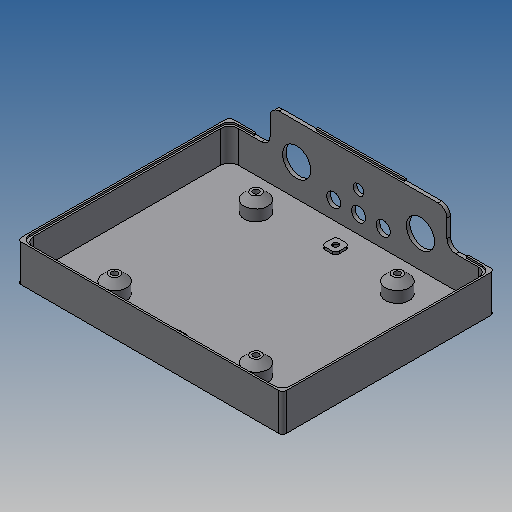
# Autodesk Inventor part: Base_Meca_IIm_Ligne
Saved by Autodesk Inventor 2025.3 (Build 293356000, 356)
## iProperties
Created: 2026-08-21
Part Number: Base_Meca_IIm_Ligne
Project: Nom Projet
Material: .
Description: Nom pièce
Document SubType Name: Modeling
Designer: jules
Authority: brut Ø
Density: 0.001 g/cm^3
Appearance: Par défaut
Mass: 0.0628592 g
Surface Area: 622.043 cm^2
Volume: 62.8592 cm^3
Material number: ---
Author: jules
Autodesk Inventor part; units mm, degrees
ref_plane "Plan YZ" through (0, 0, 0) normal (1, 0, 0) x (0, 1, 0)
ref_plane "Plan XZ" through (0, 0, 0) normal (0, 1, 0) x (-1, 0, 0)
ref_plane "Plan XY" through (0, 0, 0) normal (0, 0, 1) x (1, 0, 0)
sketch "Esquisse1" plane through (0, 0, 0) normal (0, 0, 1) x (1, 0, 0)
  line L0 (40, -40) -> (-40, -40) construction
  line L1 (-40, -40) -> (-40, 40) construction
  line L2 (-40, 40) -> (40, 40) construction
  line L3 (40, 40) -> (40, -40) construction
  line L4 (40, -40) -> (-40, 40) construction
  line L5 (-40, -40) -> (40, 40) construction
  line L6 (75, -60) -> (-75, -60)
  line L7 (-75, -60) -> (-75, 60)
  line L8 (-75, 60) -> (75, 60)
  line L9 (75, 60) -> (75, -60)
  line L10 (75, -60) -> (-75, 60) construction
  line L11 (-75, -60) -> (75, 60) construction
  line L12 (-36.8246, 40) -> (-38.4123, 37.25)
  line L13 (-38.4123, 37.25) -> (-41.5877, 37.25)
  line L14 (-41.5877, 37.25) -> (-43.1754, 40)
  line L15 (-43.1754, 40) -> (-41.5877, 42.75)
  line L16 (-41.5877, 42.75) -> (-38.4123, 42.75)
  line L17 (-38.4123, 42.75) -> (-36.8246, 40)
  line L18 (0, -84) -> (0, 84) construction
  line L19 (-105, 0) -> (105, 0) construction
  circle A0 centre (-40, 40) radius 1.75 construction
  circle A1 centre (-40, 40) radius 6.75
  line L20 (43.1754, 40) -> (41.5877, 37.25)
  line L21 (41.5877, 42.75) -> (43.1754, 40)
  line L22 (38.4123, 42.75) -> (41.5877, 42.75)
  line L23 (36.8246, 40) -> (38.4123, 42.75)
  line L24 (38.4123, 37.25) -> (36.8246, 40)
  line L25 (41.5877, 37.25) -> (38.4123, 37.25)
  circle A2 centre (40, 40) radius 6.75
  line L26 (-36.8246, -40) -> (-38.4123, -42.75)
  line L27 (-38.4123, -37.25) -> (-36.8246, -40)
  line L28 (-41.5877, -37.25) -> (-38.4123, -37.25)
  line L29 (-43.1754, -40) -> (-41.5877, -37.25)
  line L30 (-41.5877, -42.75) -> (-43.1754, -40)
  line L31 (-38.4123, -42.75) -> (-41.5877, -42.75)
  circle A3 centre (-40, -40) radius 6.75
  line L32 (43.1754, -40) -> (41.5877, -42.75)
  line L33 (41.5877, -37.25) -> (43.1754, -40)
  line L34 (38.4123, -37.25) -> (41.5877, -37.25)
  line L35 (36.8246, -40) -> (38.4123, -37.25)
  line L36 (38.4123, -42.75) -> (36.8246, -40)
  line L37 (41.5877, -42.75) -> (38.4123, -42.75)
  circle A4 centre (40, -40) radius 6.75
  circle A5 centre (0, 45.025) radius 1.6 construction
  circle A6 centre (0, -45.025) radius 1.6 construction
  line L38 (-2.75, 46.6127) -> (0, 48.2004)
  line L39 (0, 48.2004) -> (2.75, 46.6127)
  line L40 (2.75, 46.6127) -> (2.75, 43.4373)
  line L41 (2.75, 43.4373) -> (0, 41.8496)
  line L42 (0, 41.8496) -> (-2.75, 43.4373)
  line L43 (-2.75, 43.4373) -> (-2.75, 46.6127)
  line L44 (-2.75, -46.6127) -> (0, -48.2004)
  line L45 (0, -48.2004) -> (2.75, -46.6127)
  line L46 (2.75, -46.6127) -> (2.75, -43.4373)
  line L47 (2.75, -43.4373) -> (0, -41.8496)
  line L48 (0, -41.8496) -> (-2.75, -43.4373)
  line L49 (-2.75, -43.4373) -> (-2.75, -46.6127)
  point P0 (0, 0)
  dimension "d0" = 80
  dimension "d1" = 80
  dimension "d2" = 150
  dimension "d3" = 120
  dimension "d7" = 5.5
  dimension "d9" = 3.5
  dimension "d10" = 5
  dimension "d13" = 80
  dimension "d16" = 80
  dimension "d73" = 3.2
  dimension "d74" = 90.05
  dimension "d75" = 5.5
  constraints: 96 end point, 7 centre point, 7 symmetric about line, 4 coincident, 4 midpoint, 4 parallel, 3 horizontal, 3 point on line, 2 perpendicular, 1 vertical, 69 other
  measures "d0" distance of L1.end L2.end
  measures "d1" distance of L0.end L1.end
  measures "d2" distance of L7.end L8.end
  measures "d3" distance of L6.end L7.end
  measures "d7" distance between parallel lines of L13 L16
  measures "d9" diameter of A0
  measures "d10" radial gap between concentric circles of A1 A0
  measures "d13" distance of L12.start L20.start
  measures "d16" distance of L12.start L26.start
  measures "d73" diameter of A5
  measures "d74" distance of A6.centre A5.centre
  measures "d75" distance between parallel lines of L40 L43
extrude "Extrusion1" add sketch "Esquisse1" along normal blind 20 contours L6 L7 L8 L9 | L12 L13 L14 L15 L16 L17 | A1 | L20 L25 L24 L23 L22 L21 | A2 | L26 L31 L30 L29 L28 L27 | A3 | L32 L37 L36 L35 L34 L33 | A4 | L38 L39 L40 L41 L42 L43 | L49 L48 L47 L46 L45 L44
shell "Coque1" thickness 2 removed faces 1 at (-25, 20, 20)
extrude "Extrusion2" add sketch "Esquisse1" along normal blind 12 contours L12 L13 L14 L15 L16 L17 | A1 | L20 L25 L24 L23 L22 L21 | A2 | L26 L31 L30 L29 L28 L27 | A3 | L32 L37 L36 L35 L34 L33 | A4
hole "Perçage1" at (-40, -40, 0) at (40, -40, 0) at (-40, 40, 0) at (40, 40, 0) direction (0, 0, 1) diameter 3.4 end through all start extended yes clearance for "Vis à tête plate fraisée ISO 2009/7046" size "M3" standard "ISO"
extrude "Extrusion3" cut sketch "Esquisse1" along normal blind 4 contours L12 L13 L14 L15 L16 L17 | L20 L25 L24 L23 L22 L21 | L26 L31 L30 L29 L28 L27 | L32 L37 L36 L35 L34 L33
chamfer "Chanfrein1" distance 3.75 angle 45 1 edges at (-46.75, -40, 12)
chamfer "Chanfrein2" distance 3.75 angle 45 3 edges at (-46.75, 40, 12) (33.25, 40, 12) (33.25, -40, 12)
sketch "Esquisse6" plane through (-75, 60, 0) normal (0, 1, 0) x (1, 0, 0)
  line L0 (150, 0) -> (150, -20) construction
  line L1 (150, -20) -> (0, -20) projected
  line L2 (0, 0) -> (0, -20) construction
  line L3 (0, 0) -> (150, 0) construction
  line L4 (75, 8) -> (75, -48) construction
  line L5 (125, -20) -> (125, -40)
  line L6 (125, -40) -> (25, -40)
  line L7 (25, -40) -> (25, -20)
  circle A0 centre (110, -20) radius 8 construction
  circle A1 centre (40, -20) radius 8 construction
  circle A2 centre (75, -12) radius 4 construction
  circle A3 centre (75, -12) radius 5.5 construction
  circle A4 centre (89, -12) radius 4 construction
  circle A5 centre (89, -12) radius 5.5 construction
  line L8 (89, -12) -> (61, -12) construction
  circle A6 centre (61, -12) radius 4 construction
  circle A7 centre (61, -12) radius 5.5 construction
  circle A8 centre (75, -24) radius 3.25 construction
  point P0 (75, 0)
  dimension "d36" = 20
  dimension "d37" = 50
  dimension "d38" = 50
  dimension "d41" = 16
  dimension "d42" = 35
  dimension "d43" = 8
  dimension "d44" = 12
  dimension "d45" = 11
  dimension "d46" = 8
  dimension "d47" = 11
  dimension "d48" = 28
  dimension "d49" = 6.5
  dimension "d50" = 12
  constraints: 9 centre point, 8 end point, 5 point on line, 3 coincident, 2 perpendicular, 2 symmetric about line, 1 horizontal, 1 midpoint, 1 vertical, 3 other
  measures "d36" distance of L5.start L5.end
  measures "d37" distance between parallel lines of L7 L4
  measures "d38" distance between parallel lines of L5 L4
  measures "d41" diameter of A0
  measures "d42" distance from line of L4 A0.centre
  measures "d43" diameter of A2
  measures "d44" distance from line of A2.centre L3
  measures "d45" diameter of A3
  measures "d46" diameter of A4
  measures "d47" diameter of A5
  measures "d48" distance of L8.end A4.centre
  measures "d49" diameter of A8
  measures "d50" distance of A3.centre A8.centre
extrude "Extrusion4" add sketch "Esquisse6" against normal up to surface (2 mm away)
hole "Perçage2" at (-35, 60, 20) at (35, 60, 20) direction (0, -1, 0) diameter 16 depth 2 tip angle 118 start extended yes
hole "Perçage3" at (14, 60, 12) at (0, 60, 12) at (-14, 60, 12) direction (0, -1, 0) diameter 8 depth 2 tip angle 118 start extended yes
hole "Perçage4" at (0, 60, 24) direction (0, -1, 0) diameter 6 depth 10 tip angle 118 start extended yes
fillet "Congé1" radius 5 4 edges at (50, 59, 20) (50, 59, 40) (-50, 59, 40) (-50, 59, 20)
fillet "Congé2" radius 5 4 edges at (-73, 58, 11) (73, 58, 11) (73, -58, 11) (-73, -58, 11)
sketch "Esquisse7" plane through (0, 0, 20) normal (0, 0, 1) x (1, 0, 0)
  line L0 (75, 60) -> (55, 60) projected
  line L1 (75, -60) -> (75, 60) projected
  line L2 (-75, -60) -> (75, -60) projected
  line L3 (-75, 60) -> (-75, -60) projected
  line L4 (-55, 60) -> (-75, 60) projected
  line L5 (60, 60) -> (60, 59)
  line L6 (60, 59) -> (74, 59)
  line L7 (74, 59) -> (74, -59)
  line L8 (74, -59) -> (0, -59)
  line L9 (0, -84) -> (0, 84) construction
  line L10 (-60, 60) -> (-60, 59)
  line L11 (-60, 59) -> (-74, 59)
  line L12 (-74, 59) -> (-74, -59)
  line L13 (-74, -59) -> (0, -59)
  point P0 (0, 0)
  dimension "d85" = 1
  dimension "d86" = 1
  dimension "d87" = 1
  dimension "d88" = 15
  constraints: 16 end point, 4 symmetric about line, 1 horizontal, 1 parallel, 1 perpendicular, 1 point on line, 1 vertical
  measures "d85" distance of L5.start L5.end
  measures "d86" distance between parallel lines of L2 L8
  measures "d87" distance between parallel lines of L1 L7
  measures "d88" distance between parallel lines of L1 L5
extrude "Extrusion5" add sketch "Esquisse7" along normal blind 1
fillet "Congé4" radius 2 4 edges at (-75, 60, 10.5) (-75, -60, 10.5) (75, -60, 10.5) (75, 60, 10.5)
fillet "Congé5" radius 5 4 edges at (-74, 59, 20.5) (-74, -59, 20.5) (74, -59, 20.5) (74, 59, 20.5)
sketch "Esquisse8" plane through (-45, 60, 40) normal (0, 0, 1) x (1, 0, 0)
  line L0 (0, 0) -> (90, 0) projected
  line L1 (45, -144) -> (45, 24) construction
  line L2 (70, 0) -> (70, -1)
  line L3 (70, -1) -> (45, -1)
  line L4 (20, 0) -> (20, -1)
  line L5 (20, -1) -> (45, -1)
  point P0 (45, -60)
  dimension "d93" = 1
  dimension "d94" = 50
  constraints: 8 end point, 3 symmetric about line, 2 perpendicular, 2 point on line
  measures "d93" distance of L2.start L2.end
  measures "d94" distance between parallel lines of L2 L4
extrude "Extrusion6" add sketch "Esquisse8" along normal blind 1
sketch "Esquisse9" plane through (-68, -58, 2) normal (0, 0, 1) x (1, 0, 0)
  line L0 (68, -26) -> (68, 142) construction
  line L1 (64, 107.025) -> (72, 107.025)
  line L2 (72, 107.025) -> (72, 99.025)
  line L3 (72, 99.025) -> (64, 99.025)
  line L4 (64, 99.025) -> (64, 107.025)
  line L5 (64, 107.025) -> (72, 99.025) construction
  line L6 (72, 107.025) -> (64, 99.025) construction
  line L7 (-37, 58) -> (173, 58) construction
  line L8 (64, 8.975) -> (72, 8.975)
  line L9 (72, 8.975) -> (72, 16.975)
  line L10 (72, 16.975) -> (64, 16.975)
  line L11 (64, 16.975) -> (64, 8.975)
  point P0 (68, 58)
  point P1 (68, 103.025)
  dimension "d97" = 8
  dimension "d98" = 8
  constraints: 20 end point, 4 symmetric about line, 2 midpoint, 2 parallel, 1 horizontal, 1 perpendicular
  measures "d97" distance of L2.end L3.end
  measures "d98" distance of L1.end L2.end
extrude "Extrusion7" add sketch "Esquisse9" along normal blind 1.45
hole "Perçage5" at (0, -45.025, 0) at (0, 45.025, 0) direction (0, 0, 1) diameter 3.4 end through all start extended yes clearance for "Vis d'assemblage à tête hexagonale ISO 24017" size "M3" standard "ISO"
fillet "Congé6" radius 2 8 edges at (-4, -41.025, 2.725) (-4, -49.025, 2.725) (4, -41.025, 2.725) (4, 41.025, 2.725) (-4, 41.025, 2.725) (4, 49.025, 2.725) (4, -49.025, 2.725) (-4, 49.025, 2.725)
extrude "Extrusion8" cut sketch "Esquisse1" along normal blind 2.6 contours L38 L39 L40 L41 L42 L43 | L49 L48 L47 L46 L45 L44
equation "\"d13\" = d0"
equation "\"d16\" = d1"
equation "\"d38\" = d37"
